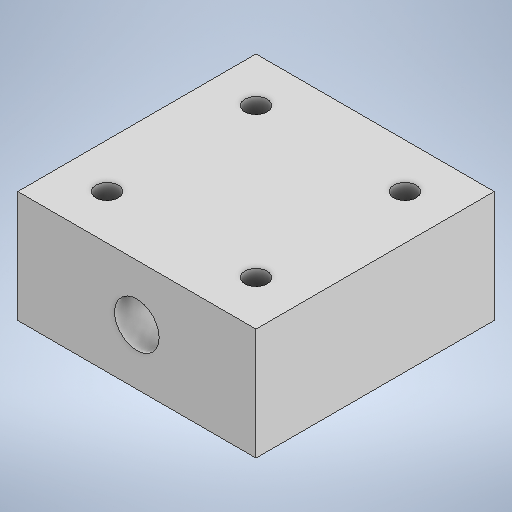
# Autodesk Inventor part: AE_MOVING_STAGE
Saved by Autodesk Inventor 2025.2 (Build 292293000, 293)
## iProperties
Created: 2026-02-09
Part Number: AE_MOVING_STAGE
Material: Generic
Document SubType Name: Modeling
Designer: composite
Density: 1 g/cm^3
Appearance: Default
Author: composite
Autodesk Inventor part; units mm, degrees
ref_plane "YZ Plane" through (0, 0, 0) normal (1, 0, 0) x (0, 1, 0)
ref_plane "XZ Plane" through (0, 0, 0) normal (0, 1, 0) x (-1, 0, 0)
ref_plane "XY Plane" through (0, 0, 0) normal (0, 0, 1) x (1, 0, 0)
sketch "Sketch1" plane through (0, 0, 0) normal (0, 1, 0) x (-1, 0, 0)
  line L0 (0, 0) -> (32, 0)
  line L1 (32, 0) -> (32, -32)
  line L2 (32, -32) -> (0, -32)
  line L3 (0, -32) -> (0, 0)
  dimension "d0" = 32
  dimension "d1" = 32
  constraints: 8 end point, 2 parallel, 1 horizontal, 1 perpendicular
  measures "d0" distance of L1.end L2.end
  measures "d1" distance of L0.end L1.end
extrude "Extrusion1" add sketch "Sketch1" along normal blind 15
sketch "Sketch2" plane through (-32, 0, 0) normal (0, 0, 1) x (1, 0, 0)
  line L0 (32, 15) -> (0, 15) projected
  line L1 (0, 15) -> (32, 0) construction
  line L2 (32, 0) -> (0, 0) projected
  line L3 (0, 0) -> (32, 15) construction
  circle A0 centre (16, 7.5) radius 3
  dimension "d4" = 6
  constraints: 4 end point, 1 centre point, 1 midpoint
  measures "d4" diameter of A0
extrude "Extrusion2" cut sketch "Sketch2" against normal through all
sketch "Sketch3" plane through (0, 15, 0) normal (0, 1, 0) x (1, 0, 0)
  circle A0 centre (-26, 6) radius 1.5
  circle A1 centre (-26, 26) radius 1.5
  circle A2 centre (-6, 6) radius 1.5
  circle A3 centre (-6, 26) radius 1.5
  line L0 (-32, 0) -> (0, 0) projected
  line L1 (-32, 32) -> (-32, 0) projected
  dimension "d7" = 3
  dimension "d8" = 6
  dimension "d9" = 20
  dimension "d10" = 20
  dimension "d11" = 6
  constraints: 4 centre point, 3 equal radius, 2 horizontal alignment, 2 vertical alignment
  measures "d7" diameter of A0
  measures "d8" distance from line of L0 A0.centre
  measures "d9" distance of A1.centre A0.centre
  measures "d10" distance of A3.centre A1.centre
  measures "d11" distance from line of L1 A1.centre
extrude "Extrusion3" cut sketch "Sketch3" against normal blind 10
body "Solid1"
